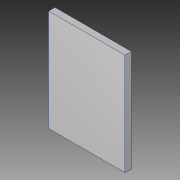
# Autodesk Inventor part: BLOCK_PLATE
Saved by Autodesk Inventor 2019 (Build 230136000, 136)
## iProperties
Created: 2019-09-01
Part Number: BLOCK_PLATE
Material: Aluminum 6061
Document SubType Name: Modeling
Designer: brand
Density: 2.7 g/cm^3
Appearance: Aluminum - Flat
Mass: 132.735 g
Surface Area: 177.419 cm^2
Volume: 49.1612 cm^3
RuleStatus: InUse
AfterDocNew0: SHOW
AfterDocOpen0: SHOW
Author: brand
Autodesk Inventor part; units mm, degrees
ref_plane "YZ Plane" through (0, 0, 0) normal (1, 0, 0) x (0, 1, 0)
ref_plane "XZ Plane" through (0, 0, 0) normal (0, 1, 0) x (-1, 0, 0)
ref_plane "XY Plane" through (0, 0, 0) normal (0, 0, 1) x (1, 0, 0)
sketch "Sketch1" plane through (0, 0, 0) normal (0, 0, 1) x (1, 0, 0)
  line L0 (-38.1, -50.8) -> (38.1, -50.8)
  line L1 (38.1, -50.8) -> (38.1, 50.8)
  line L2 (38.1, 50.8) -> (-38.1, 50.8)
  line L3 (-38.1, 50.8) -> (-38.1, -50.8)
  line L4 (-38.1, -50.8) -> (38.1, 50.8) construction
  line L5 (38.1, -50.8) -> (-38.1, 50.8) construction
  point P0 (0, 0)
  dimension "width" = 76.2
  dimension "length" = 101.6
  constraints: 12 end point, 2 midpoint, 2 parallel, 1 horizontal, 1 perpendicular
  measures "width" distance of L2.end L1.end
  measures "length" distance of L0.end L1.end
extrude "Extrusion1" add sketch "Sketch1" along normal mid plane 6.35
body "Solid1"
